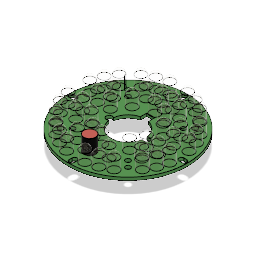
48led-ir-illuminator (Autodesk Fusion 360 design; units mm, degrees)
Autodesk Fusion 360 part; units mm, degrees
sketch "PCB outline and mounting" plane through (0, 0, 0) normal (0, 1, 0) x (1, 0, 0)
  circle A0 centre (0, 0) radius 30.15
  circle A1 centre (0, 0) radius 8.5
  line L0 (-2, 11.5) -> (2, 11.5)
  line L1 (2, 11.5) -> (2, 8.2614)
  line L2 (2, 8.2614) -> (-2, 8.2614) construction
  line L3 (-2, 8.2614) -> (-2, 11.5)
  line L4 (0, 11.5) -> (0, -8.5) construction
  circle A2 centre (-9.5, 0) radius 1.5
  circle A3 centre (9.5, 0) radius 1.5
  line L5 (-9.5, 0) -> (9.5, 0)
  line L6 (-11, 4.4079) -> (-11, 0) construction
  line L7 (11, 0) -> (11, 5) construction
  line L8 (-11, 0) -> (11, 0)
  circle A4 centre (27, 0) radius 1.25
  circle A5 centre (28.5, 0) radius 1.25
  line L9 (27, 1.25) -> (28.5, 1.25)
  line L10 (28.5, -1.25) -> (27, -1.25)
  line L11 (25.75, 0) -> (29.75, 0) construction
  line L12 (-27, -1.25) -> (-28.5, -1.25)
  circle A6 centre (-27, 0) radius 1.25
  line L13 (-29.75, 0) -> (-25.75, 0) construction
  line L14 (-28.5, 1.25) -> (-27, 1.25)
  circle A7 centre (-28.5, 0) radius 1.25
  line L15 (-1.25, -28.5) -> (-1.25, -27)
  circle A8 centre (0, -28.5) radius 1.25
  line L16 (0, -25.75) -> (0, -29.75) construction
  line L17 (1.25, -27) -> (1.25, -28.5)
  circle A9 centre (0, -27) radius 1.25
  circle A10 centre (0, 27) radius 1.25
  line L18 (0, 29.75) -> (0, 25.75) construction
  line L19 (1.25, 28.5) -> (1.25, 27)
  line L20 (-1.25, 27) -> (-1.25, 28.5)
  circle A11 centre (0, 28.5) radius 1.25
  circle A12 centre (0, 0) radius 28.5 construction
  circle A13 centre (0, 0) radius 27 construction
  line L21 (27, 0) -> (-27, 0) construction
  line L22 (0, 27) -> (0, -27) construction
  line L23 (-14, 14) -> (14, 14) construction
  line L24 (14, 14) -> (14, -14) construction
  line L25 (14, -14) -> (-14, -14) construction
  line L26 (-14, -14) -> (-14, 14) construction
  line L27 (-17, 17) -> (17, 17) construction
  line L28 (17, 17) -> (17, -17) construction
  line L29 (17, -17) -> (-17, -17) construction
  line L30 (-17, -17) -> (-17, 17) construction
  line L31 (-17, 0) -> (17, 0) construction
  line L32 (-14, 0) -> (14, 0) construction
  circle A14 centre (-17, 17) radius 1.25
  circle A15 centre (-17, -17) radius 1.25
  circle A16 centre (-14, -14) radius 1.25
  circle A17 centre (-14, 14) radius 1.25
  circle A18 centre (17, 17) radius 1.25
  circle A19 centre (14, 14) radius 1.25
  circle A20 centre (17, -17) radius 1.25
  circle A21 centre (14, -14) radius 1.25
  dimension "d1" = 17
  dimension "d2" = 60.3
  dimension "d3" = 4
  dimension "d4" = 20
  dimension "d6" = 3
  dimension "d7" = 22
  dimension "d8" = 2.5
  dimension "d9" = 4
  dimension "d10" = 2.5
  dimension "d11" = 4
  dimension "d12" = 2.5
  dimension "d13" = 4
  dimension "d14" = 2.5
  dimension "d15" = 4
  dimension "d16" = 54
  dimension "d17" = 57
  dimension "d18" = 28
  dimension "d19" = 34
  dimension "d20" = 2.5
  measures "d1" diameter of A1
  measures "d2" diameter of A0
  measures "d6" diameter of A3
  measures "d8" diameter of A4
  measures "d10" diameter of A7
  measures "d12" diameter of A9
  measures "d14" diameter of A11
  measures "d16" diameter of A13
  measures "d17" diameter of A12
  measures "d20" diameter of A14
extrude "Extrude1" add sketch "PCB outline and mounting" along normal blind 1.56 makes body 1
sketch "Front components" plane through (0, 1.56, 0) normal (0, 1, 0) x (-1, 0, 0)
  circle A0 centre (-14, 14) radius 1.25
  circle A1 centre (-14, -14) radius 1.25
  circle A2 centre (-17, 17) radius 1.25
  circle A3 centre (17, -17) radius 1.25
  circle A4 centre (-17, -17) radius 1.25
  circle A5 centre (17, 17) radius 1.25
  circle A6 centre (14, 14) radius 1.25
  circle A7 centre (14, -14) radius 1.25
  arc A8 (1.25, -27) -> (-1.25, -27) centre (0, -27) ccw
  line L0 (1.25, -27) -> (1.25, -28.5)
  arc A9 (-1.25, -28.5) -> (1.25, -28.5) centre (0, -28.5) ccw
  line L1 (-1.25, -28.5) -> (-1.25, -27)
  arc A10 (1.25, 28.5) -> (-1.25, 28.5) centre (0, 28.5) ccw
  line L2 (1.25, 28.5) -> (1.25, 27)
  arc A11 (-1.25, 27) -> (1.25, 27) centre (0, 27) ccw
  line L3 (-1.25, 27) -> (-1.25, 28.5)
  arc A12 (28.5, -1.25) -> (28.5, 1.25) centre (28.5, 0) ccw
  line L4 (28.5, -1.25) -> (27, -1.25)
  arc A13 (27, 1.25) -> (27, -1.25) centre (27, 0) ccw
  line L5 (27, 1.25) -> (28.5, 1.25)
  arc A14 (-27, -1.25) -> (-27, 1.25) centre (-27, 0) ccw
  line L6 (-27, -1.25) -> (-28.5, -1.25)
  arc A15 (-28.5, 1.25) -> (-28.5, -1.25) centre (-28.5, 0) ccw
  line L7 (-28.5, 1.25) -> (-27, 1.25)
  arc A16 (2, -8.2614) -> (8.4342, -1.0555) centre (0, 0) ccw
  line L8 (2, -8.2614) -> (2, -11.5)
  line L9 (2, -11.5) -> (-2, -11.5)
  line L10 (-2, -11.5) -> (-2, -8.2614)
  arc A17 (-8.4342, -1.0555) -> (-2, -8.2614) centre (0, 0) ccw
  arc A18 (-8.4342, 1.0555) -> (-8.4342, -1.0555) centre (-9.5, 0) ccw
  arc A19 (8.4342, 1.0555) -> (-8.4342, 1.0555) centre (0, 0) ccw
  arc A20 (8.4342, -1.0555) -> (8.4342, 1.0555) centre (9.5, 0) ccw
  circle A21 centre (0, 0) radius 30.15
  circle A22 centre (0, 0) radius 13.5 construction
  circle A23 centre (0, 0) radius 19.5 construction
  circle A24 centre (0, 0) radius 26 construction
  circle A25 centre (-0.1186, 19.4996) radius 3
  circle A26 centre (5.5997, 25.3898) radius 2.5
  circle A27 centre (10.9897, 23.5633) radius 2.5
  circle A28 centre (15.5545, 20.834) radius 2.5
  circle A29 centre (20.5895, 15.8768) radius 2.5
  circle A30 centre (23.8466, 10.3605) radius 2.5
  circle A31 centre (25.5847, 4.6284) radius 2.5
  circle A32 centre (7.545, 17.9812) radius 2.5
  circle A33 centre (-8.1407, 17.7195) radius 2.5
  circle A34 centre (-16.8081, 9.8862) radius 2.5
  circle A35 centre (-19.1274, 3.7937) radius 2.5
  circle A36 centre (-19.1274, -3.7937) radius 2.5
  circle A37 centre (-17.031, -9.4971) radius 2.5
  circle A38 centre (-3.9306, 25.7012) radius 2.5
  circle A39 centre (-9.5126, 24.1973) radius 2.5
  circle A40 centre (-14.5026, 21.5795) radius 2.5
  circle A41 centre (-21.6485, 14.3994) radius 2.5
  circle A42 centre (-24.1253, 9.6939) radius 2.5
  circle A43 centre (-25.5848, 4.6278) radius 2.5
  circle A44 centre (-25.4341, -5.395) radius 2.5
  circle A45 centre (-23.6357, -10.833) radius 2.5
  circle A46 centre (-21.0369, -15.279) radius 2.5
  circle A47 centre (-14.7631, -21.4021) radius 2.5
  circle A48 centre (-9.9637, -24.0151) radius 2.5
  circle A49 centre (-4.4475, -25.6168) radius 2.5
  circle A50 centre (4.4475, -25.6168) radius 2.5
  circle A51 centre (9.9876, -24.0052) radius 2.5
  circle A52 centre (14.8208, -21.3622) radius 2.5
  circle A53 centre (20.4661, -16.0355) radius 2.5
  circle A54 centre (23.3917, -11.3503) radius 2.5
  circle A55 centre (25.3052, -5.9705) radius 2.5
  circle A56 centre (2.3645, -19.3561) radius 2.5
  circle A57 centre (-3.084, -19.2546) radius 2.5
  circle A58 centre (-8.4919, -17.5539) radius 2.5
  circle A59 centre (8.4342, -17.5816) radius 2.5
  circle A60 centre (-0.126, -13.4994) radius 2.5
  circle A61 centre (-6.5031, -11.8304) radius 2.5
  circle A62 centre (-12.4159, -5.3006) radius 2.5
  circle A63 centre (-12.9842, 3.6959) radius 2.5
  circle A64 centre (-9.9445, 9.13) radius 2.5
  circle A65 centre (-0.1954, 13.4986) radius 2.5
  circle A66 centre (5.3065, 12.4133) radius 2.5
  circle A67 centre (11.5009, 7.0695) radius 2.5
  circle A68 centre (12.9039, -3.9673) radius 2.5
  circle A69 centre (8.4342, -10.5411) radius 2.5
  circle A70 centre (17.2554, 9.083) radius 2.5
  circle A71 centre (19.1282, 3.7897) radius 2.5
  circle A72 centre (19.1282, -3.7897) radius 2.5
  circle A73 centre (16.954, -9.6339) radius 2.5
  dimension "d23" = 27
  dimension "d24" = 39
  dimension "d25" = 52
  dimension "d26" = 6
  dimension "d27" = 5
  measures "d23" diameter of A22
  measures "d24" diameter of A23
  measures "d25" diameter of A24
  measures "d26" diameter of A25
  measures "d27" diameter of A26
extrude "Extrude2" add sketch "Front components" along normal blind 8 separate body contours A3 A53 | L9 A60 | L9 A60 | A26 | A27 | A28 | A29 | A30 | A31 | A32 | A33 | A34 | A35 | A36 | A37 | A38 | A39 | A40 | A41 | A42 | A43 | A44 | A45 | A46 | A47 | A48 | A49 | A50 | A51 | A52 | A54 | A55 | A56 | A57 | A58 | A59 | A61 | A62 | A63 | A64 | A65 | A66 | A67 | A68 | A69 | A70 | A71 | A72 | A73 picked at (21.3696, -16.3684) makes body 2 at (7.4476, 6.8933, 9.0054) makes body 3 at (21.6284, 6.8933, 9.5692) makes body 4 at (1.4337, 6.8933, 25.5766) makes body 5 at (-10.0419, 6.8933, 17.8566) makes body 6 at (-23.0864, 6.8933, 15.7522) makes body 7 at (-13.9978, 6.8933, 6.9449) makes body 8 at (-21.6251, 6.8933, -3.9143) makes body 9 at (-10.9311, 6.8933, -17.7063) makes body 10 at (4.0062, 6.8933, -11.9551) makes body 11 at (22.9372, 6.8933, -5.5196) makes body 12 at (7.4669, 6.8933, -24.1397) makes body 13 at (-17.3176, 6.8933, -21.4869) makes body 14 at (-12.4845, 6.8933, -24.1298) makes body 15 at (12.2662, 6.8933, -21.5267) makes body 16 at (16.6305, 6.8933, -3.9183) makes body 17 at (5.995, 6.8933, -17.6785) makes body 18 at (-10.9311, 6.8933, -10.6657) makes body 19 at (-27.8021, 6.8933, -6.0951) makes body 20 at (-19.7523, 6.8933, 8.9584) makes body 21 at (-18.0514, 6.8933, 20.7094) makes body 22 at (-7.8034, 6.8933, 12.2887) makes body 23 at (7.0157, 6.8933, 24.0727) makes body 24 at (23.0879, 6.8933, 4.5032) makes body 25 at (10.4873, 6.8933, 3.5713) makes body 26 at (14.3112, 6.8933, 9.7616) makes body 27 at (19.1516, 6.8933, 14.2748) makes body 28 at (5.6438, 6.8933, 17.5948) makes body 29 at (-8.0966, 6.8933, 25.2652) makes body 30 at (-28.0816, 6.8933, 4.5038) makes body 31 at (-21.6251, 6.8933, 3.6651) makes body 32 at (-19.4509, 6.8933, -9.7585) makes body 33 at (-4.8614, 6.8933, -19.4807) makes body 34 at (9.919, 6.8933, -5.4252) makes body 35 at (21.1388, 6.8933, -10.9576) makes body 36 at (1.9506, 6.8933, -25.7414) makes body 37 at (-21.1405, 4.2267, -18.4428) makes body 38 at (-6.9443, 6.8933, -25.7414) makes body 39 at (18.54, 6.8933, -15.4036) makes body 40 at (14.5341, 6.8933, -9.6217) makes body 41 at (0.5872, 6.8933, -19.3792) makes body 42 at (-15.4008, 6.8933, -4.0919) makes body 43 at (-25.8886, 6.8933, -11.4749) makes body 44 at (-26.3435, 6.8933, 10.2359) makes body 45 at (-13.4866, 6.8933, 23.4386) makes body 46 at (-2.3015, 6.8933, 13.374) makes body 47 at (12.0057, 6.8933, 21.4549) makes body 48 at (16.6305, 6.8933, 3.669) makes body 49 at (-2.3616, 6.8933, -13.2505)
fillet "Fillet1" radius 2.5 48 edges at (12.2753, 9.56, 8.2259) (26.4561, 9.56, 8.7898) (6.2614, 9.56, 24.7971) (-5.2142, 9.56, 17.0772) (-18.2587, 9.56, 14.9727) (-9.1701, 9.56, 6.1655) (-16.7974, 9.56, -4.6938) (-6.1034, 9.56, -18.4857) (8.8339, 9.56, -12.7345) (27.7649, 9.56, -6.299) (12.2946, 9.56, -24.9191) (-12.4899, 9.56, -22.2663) (-7.6568, 9.56, -24.9092) (17.0939, 9.56, -22.3062) (21.4582, 9.56, -4.6977) (10.8227, 9.56, -18.4579) (-6.1034, 9.56, -11.4451) (-22.9744, 9.56, -6.8745) (-14.9246, 9.56, 8.179) (-13.2237, 9.56, 19.93) (-2.9757, 9.56, 11.5093) (11.8434, 9.56, 23.2933) (27.9156, 9.56, 3.7238) (15.3151, 9.56, 2.7918) (19.139, 9.56, 8.9821) (23.9793, 9.56, 13.4954) (10.4715, 9.56, 16.8154) (-3.2689, 9.56, 24.4858) (-23.2539, 9.56, 3.7244) (-16.7974, 9.56, 2.8857) (-14.6232, 9.56, -10.5379) (-0.0337, 9.56, -20.2602) (14.7467, 9.56, -6.2046) (25.9665, 9.56, -11.7371) (6.7783, 9.56, -26.5208) (-22.8746, 9.56, -15.3653) (-2.1166, 9.56, -26.5208) (23.3678, 9.56, -16.183) (19.3618, 9.56, -10.4011) (5.4149, 9.56, -20.1586) (-10.5731, 9.56, -4.8713) (-21.0609, 9.56, -12.2543) (-21.5158, 9.56, 9.4565) (-8.6588, 9.56, 22.6592) (2.5262, 9.56, 12.5945) (16.8334, 9.56, 20.6755) (21.4582, 9.56, 2.8896) (2.4568, 9.56, -14.4035) on bodies 2 3 4 5 6 7 8 9 10 11 12 13 14 15 16 17 18 19 20 21 22 23 24 25 26 27 28 29 30 31 32 33 34 35 36 37 38 39 40 41 42 43 44 45 46 47 48 49
extrude "Extrude3" add sketch "Front components" along normal blind 7.5 contours A25 bodies 1
sketch "Back components" plane through (0, 0, 0) normal (0, -1, 0) x (1, 0, 0)
  circle A0 centre (14, 14) radius 1.25
  circle A1 centre (14, -14) radius 1.25
  circle A2 centre (17, 17) radius 1.25
  circle A3 centre (-17, -17) radius 1.25
  circle A4 centre (17, -17) radius 1.25
  circle A5 centre (-17, 17) radius 1.25
  circle A6 centre (-14, 14) radius 1.25
  circle A7 centre (-14, -14) radius 1.25
  arc A8 (1.25, -27) -> (-1.25, -27) centre (0, -27) ccw
  line L0 (1.25, -27) -> (1.25, -28.5)
  arc A9 (-1.25, -28.5) -> (1.25, -28.5) centre (0, -28.5) ccw
  line L1 (-1.25, -28.5) -> (-1.25, -27)
  arc A10 (1.25, 28.5) -> (-1.25, 28.5) centre (0, 28.5) ccw
  line L2 (1.25, 28.5) -> (1.25, 27)
  arc A11 (-1.25, 27) -> (1.25, 27) centre (0, 27) ccw
  line L3 (-1.25, 27) -> (-1.25, 28.5)
  arc A12 (-28.5, 1.25) -> (-28.5, -1.25) centre (-28.5, 0) ccw
  line L4 (-28.5, 1.25) -> (-27, 1.25)
  arc A13 (-27, -1.25) -> (-27, 1.25) centre (-27, 0) ccw
  line L5 (-27, -1.25) -> (-28.5, -1.25)
  arc A14 (27, 1.25) -> (27, -1.25) centre (27, 0) ccw
  line L6 (27, 1.25) -> (28.5, 1.25)
  arc A15 (28.5, -1.25) -> (28.5, 1.25) centre (28.5, 0) ccw
  line L7 (28.5, -1.25) -> (27, -1.25)
  arc A16 (-8.4342, -1.0555) -> (-2, -8.2614) centre (0, 0) ccw
  arc A17 (-8.4342, 1.0555) -> (-8.4342, -1.0555) centre (-9.5, 0) ccw
  arc A18 (8.4342, 1.0555) -> (-8.4342, 1.0555) centre (0, 0) ccw
  arc A19 (8.4342, -1.0555) -> (8.4342, 1.0555) centre (9.5, 0) ccw
  arc A20 (2, -8.2614) -> (8.4342, -1.0555) centre (0, 0) ccw
  line L8 (2, -8.2614) -> (2, -11.5)
  line L9 (2, -11.5) -> (-2, -11.5)
  line L10 (-2, -11.5) -> (-2, -8.2614)
  circle A21 centre (0, 0) radius 30.15
  line L11 (-7.9386, 22.2425) -> (-1.9386, 20.9672)
  line L12 (-1.9386, 20.9672) -> (-3.0014, 15.9672)
  line L13 (-3.0014, 15.9672) -> (-9.0014, 17.2425)
  line L14 (-9.0014, 17.2425) -> (-7.9386, 22.2425)
  circle A22 centre (-4.2, 19.1048) radius 0.625
  circle A23 centre (-6.74, 19.1048) radius 0.625
  line L15 (-6.74, 19.1048) -> (0, 19.1048) construction
  line L16 (0, 0) -> (0, 19.1048) construction
  line L17 (-6.74, 19.1048) -> (-4.2, 19.1048) construction
  line L18 (-5.47, 19.1048) -> (-8.1075, 19.6654) construction
  line L19 (-8.47, 19.7425) -> (-2.47, 18.4672) construction
  dimension "d33" = 1.25
  dimension "d34" = 4.2
  dimension "d35" = 2.54
  dimension "d36" = 6
  dimension "d37" = 5
  dimension "d38" = 12
  measures "d33" diameter of A23
  measures "d34" distance of L16
  measures "d38" angle of L15 L18
extrude "Extrude4" add sketch "Back components" along normal blind 6 contours L11 L12 L13 L14 | A22 | A23 bodies 1
named bodies: "PCB"
